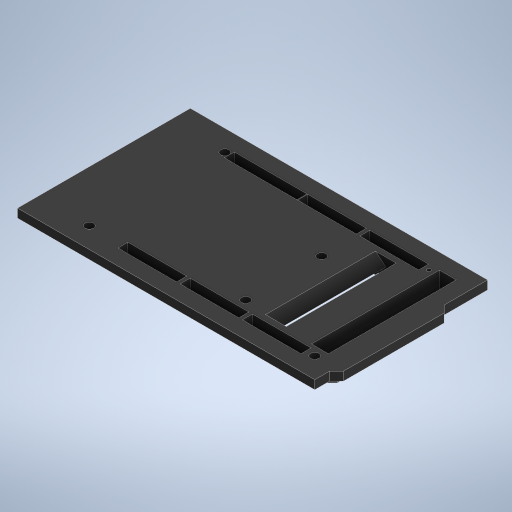
# Autodesk Inventor part: ArduinoMegaCaseTop
Saved by Autodesk Inventor 2024 (Build 280153000, 153)
## iProperties
Created: 2023-07-08
Part Number: ArduinoMegaCaseTop
Material: Rubber, Silicone
Document SubType Name: Modeling
Designer: 18179
Density: 1.25 g/cm^3
Appearance: Rubber - Black
Author: 18179
Autodesk Inventor part; units mm, degrees
ref_plane "YZ Plane" through (0, 0, 0) normal (1, 0, 0) x (0, 1, 0)
ref_plane "XZ Plane" through (0, 0, 0) normal (0, 1, 0) x (-1, 0, 0)
ref_plane "XY Plane" through (0, 0, 0) normal (0, 0, 1) x (1, 0, 0)
sketch "Sketch3" plane through (0, 0, 0) normal (0, 1, 0) x (-1, 0, 0)
  line L0 (0, 0) -> (0, -53.34)
  line L1 (0, -53.34) -> (0, -50.165)
  line L2 (0, -50.165) -> (1.905, -50.165)
  line L3 (1.905, -50.165) -> (0, -50.165)
  line L4 (0, -50.165) -> (0, -41.165)
  line L5 (0, -41.165) -> (1.905, -41.165)
  line L6 (1.905, -41.165) -> (1.905, -50.165)
  line L7 (0, 0) -> (0, -9.3)
  line L8 (0, -9.3) -> (6.35, -9.3)
  line L9 (6.35, -9.3) -> (0, -9.3)
  line L10 (0, -9.3) -> (0, -21.34)
  line L11 (0, -21.34) -> (6.35, -21.34)
  line L12 (6.35, -21.34) -> (6.35, -9.3)
  line L13 (0, -53.34) -> (-99.06, -53.34)
  line L14 (0, 0) -> (-99.06, 0)
  line L15 (0, -53.34) -> (-13.67, -53.34) construction
  line L16 (-13.67, -53.34) -> (-13.67, -50.8) construction
  line L17 (-13.67, -50.8) -> (0, -50.8) construction
  line L18 (0, -50.8) -> (0, -53.34) construction
  line L19 (0, 0) -> (-15.24, 0) construction
  line L20 (-15.24, 0) -> (-15.24, -2.54) construction
  line L21 (-15.24, -2.54) -> (0, -2.54) construction
  line L22 (0, -2.54) -> (0, 0) construction
  line L23 (-99.06, 0) -> (-90.17, 0) construction
  line L24 (-90.17, 0) -> (-90.17, -2.54) construction
  line L25 (-90.17, -2.54) -> (-99.06, -2.54) construction
  line L26 (-99.06, -2.54) -> (-99.06, 0) construction
  line L27 (-99.06, -53.34) -> (-96.52, -53.34) construction
  line L28 (-96.52, -53.34) -> (-96.52, -50.8) construction
  line L29 (-96.52, -50.8) -> (-99.06, -50.8) construction
  line L30 (-99.06, -50.8) -> (-99.06, -53.34) construction
  line L31 (-99.06, 0) -> (-66.04, 0) construction
  line L32 (-66.04, 0) -> (-66.04, -17.78) construction
  line L33 (-66.04, -17.78) -> (-99.06, -17.78) construction
  line L34 (-99.06, -17.78) -> (-99.06, 0) construction
  line L35 (-99.06, -53.34) -> (-66.04, -53.34) construction
  line L36 (-66.04, -53.34) -> (-66.04, -45.72) construction
  line L37 (-66.04, -45.72) -> (-99.06, -45.72) construction
  line L38 (-99.06, -45.72) -> (-99.06, -53.34) construction
  line L39 (-99.06, 0) -> (-99.06, -12.954)
  line L40 (-99.06, -53.34) -> (-99.06, -50.8)
  line L41 (-99.06, -50.8) -> (-101.6, -50.8) construction
  line L42 (-101.6, -50.8) -> (-101.6, -48.26) construction
  line L43 (-101.6, -48.26) -> (-99.06, -48.26) construction
  line L44 (-99.06, -48.26) -> (-99.06, -50.8) construction
  line L45 (-99.06, -12.954) -> (-101.6, -12.954) construction
  line L46 (-101.6, -12.954) -> (-101.6, -15.494) construction
  line L47 (-101.6, -15.494) -> (-99.06, -15.494) construction
  line L48 (-99.06, -15.494) -> (-99.06, -12.954) construction
  line L49 (-99.06, -12.954) -> (-101.6, -15.494)
  line L50 (-101.6, -15.494) -> (-101.6, -48.26)
  line L51 (-101.6, -48.26) -> (-99.06, -50.8)
  circle A0 centre (-13.67, -50.8) radius 1.5875
  circle A1 centre (-15.24, -2.54) radius 1.5875
  circle A2 centre (-66.04, -17.78) radius 1.5875
  circle A3 centre (-66.04, -45.72) radius 1.5875
  circle A4 centre (-96.52, -50.8) radius 1.5875
  circle A5 centre (-90.17, -2.54) radius 1.5875
  line L52 (0, -58.42) -> (-104.14, -58.42)
  line L53 (-104.14, -58.42) -> (-104.14, -52.9042)
  line L54 (-104.14, -52.9042) -> (-106.68, -50.3642)
  line L55 (-106.68, -50.3642) -> (-106.68, -13.3898)
  line L56 (-106.68, -13.3898) -> (-104.14, -10.8498)
  line L57 (-104.14, -10.8498) -> (-104.14, 5.08)
  line L58 (-104.14, 5.08) -> (0, 5.08)
  line L59 (0, -55.245) -> (-100.965, -55.245)
  line L60 (-100.965, -55.245) -> (-100.965, -51.5891)
  line L61 (-100.965, -51.5891) -> (-103.505, -49.0491)
  line L62 (-103.505, -49.0491) -> (-103.505, -14.7049)
  line L63 (-103.505, -14.7049) -> (-100.965, -12.1649)
  line L64 (-100.965, -12.1649) -> (-100.965, 1.905)
  line L65 (-100.965, 1.905) -> (0, 1.905)
  line L66 (5.08, 0) -> (5.08, -53.34)
  line L67 (1.905, 0) -> (1.905, -53.34)
  line L68 (0, -58.42) -> (5.08, -58.42)
  line L69 (5.08, -58.42) -> (5.08, -53.34)
  line L70 (1.905, -53.34) -> (1.905, -55.245)
  line L71 (1.905, -55.245) -> (0, -55.245)
  line L72 (1.905, 0) -> (1.905, 1.905)
  line L73 (1.905, 1.905) -> (0, 1.905)
  line L74 (0, 5.08) -> (5.08, 5.08)
  line L75 (5.08, 5.08) -> (5.08, 0)
  line L76 (-0.5101, -40.6549) -> (-0.5101, -50.6751)
  line L77 (-0.5101, -50.6751) -> (2.4151, -50.6751)
  line L78 (2.4151, -50.6751) -> (2.4151, -40.6549)
  line L79 (2.4151, -40.6549) -> (-0.5101, -40.6549)
  line L80 (-102.9276, -14.9441) -> (-102.9276, -48.8099)
  line L81 (-102.9276, -48.8099) -> (-100.3876, -51.3499)
  line L82 (-100.3876, -51.3499) -> (-100.3876, -54.6676)
  line L83 (-100.3876, -54.6676) -> (1.3276, -54.6676)
  line L84 (1.3276, -54.6676) -> (1.3276, -53.34)
  line L85 (1.3276, -53.34) -> (1.3276, 0)
  line L86 (1.3276, 0) -> (1.3276, 1.3276)
  line L87 (1.3276, 1.3276) -> (-100.3876, 1.3276)
  line L88 (-100.3876, 1.3276) -> (-100.3876, -12.4041)
  line L89 (-100.3876, -12.4041) -> (-102.9276, -14.9441)
  line L90 (-100.3876, -51.3499) -> (-100.965, -51.5891)
  line L91 (-100.965, -12.1649) -> (-100.3876, -12.4041)
  line L92 (1.3276, -50.6751) -> (-8.8224, -50.6751)
  line L93 (-8.8224, -50.6751) -> (-8.8224, -40.6549)
  line L94 (-8.8224, -40.6549) -> (1.3276, -40.6549)
  line L95 (1.3276, -40.6549) -> (1.3276, -50.6751)
  line L96 (0, -9.3) -> (-12.595, -9.3)
  line L97 (-12.595, -9.3) -> (-12.595, -21.34)
  line L98 (-12.595, -21.34) -> (0, -21.34)
  line L99 (0, -21.34) -> (0, -9.3)
  line L100 (0.7276, -22.0676) -> (-13.3226, -22.0676)
  line L101 (-13.3226, -22.0676) -> (-13.3226, -8.5724)
  line L102 (-13.3226, -8.5724) -> (0.7276, -8.5724)
  line L103 (0.7276, -8.5724) -> (0.7276, -22.0676)
  point P0 (5.08, -21.34)
  point P1 (1.905, -21.34)
  point P2 (1.905, -9.3)
  point P3 (5.08, -9.3)
  point P4 (0.7276, -9.3)
  point P5 (1.3276, -9.3)
  point P6 (1.3276, -40.6549)
  point P7 (1.3276, -21.34)
  point P8 (0.7276, -21.34)
  dimension "d74" = 53.34
  dimension "d75" = 3.175
  dimension "d76" = 1.905
  dimension "d77" = 9
  dimension "d78" = 9.3
  dimension "d79" = 6.35
  dimension "d80" = 12.04
  dimension "d81" = 99.06
  dimension "d82" = 99.06
  dimension "d83" = 13.67
  dimension "d84" = 2.54
  dimension "d85" = 15.24
  dimension "d86" = 2.54
  dimension "d87" = 8.89
  dimension "d88" = 2.54
  dimension "d89" = 2.54
  dimension "d90" = 2.54
  dimension "d91" = 17.78
  dimension "d92" = 33.02
  dimension "d93" = 33.02
  dimension "d94" = 7.62
  dimension "d95" = 12.954
  dimension "d96" = 2.54
  dimension "d97" = 2.54
  dimension "d98" = 2.54
  dimension "d99" = 2.54
  dimension "d100" = 2.54
  dimension "d101" = 3.175
  dimension "d102" = 3.175
  dimension "d103" = 3.175
  dimension "d104" = 3.175
  dimension "d105" = 3.175
  dimension "d106" = 3.175
  dimension "d107" = 5.08
  dimension "d108" = 3.175
  dimension "d109" = 5.08
  dimension "d110" = 3.175
  dimension "d193" = 10.15
  dimension "d194" = 12.595
  constraints: 208 end point, 31 parallel, 19 perpendicular, 16 horizontal, 9 point on line, 6 centre point, 6 coincident, 2 vertical, 1 collinear, 27 other
  measures "d74" distance of L0.start L0.end
  measures "d75" distance of L0.end L1.end
  measures "d76" distance of L1.end L2.end
  measures "d77" distance of L3.end L4.end
  measures "d78" distance of L0.start L7.end
  measures "d79" distance of L7.end L8.end
  measures "d80" distance of L10.end L9.end
  measures "d81" distance of L0.end L13.end
  measures "d82" distance of L0.start L14.end
  measures "d83" distance of L16.end L17.end
  measures "d84" distance of L15.end L16.end
  measures "d85" distance of L21.end L20.end
  measures "d86" distance of L20.end L19.end
  measures "d87" distance of L24.end L25.end
  measures "d88" distance of L23.end L24.end
  measures "d89" distance of L29.end L28.end
  measures "d90" distance of L28.end L27.end
  measures "d91" distance of L31.end L32.end
  measures "d92" distance of L32.end L33.end
  measures "d93" distance of L37.end L36.end
  measures "d94" distance of L36.end L35.end
  measures "d95" distance of L14.end L39.end
  measures "d96" distance of L13.end L29.end
  measures "d97" distance of L42.end L43.end
  measures "d98" distance of L41.end L42.end
  measures "d99" distance of L47.end L46.end
  measures "d100" distance of L46.end L45.end
  measures "d101" diameter of A0
  measures "d102" diameter of A1
  measures "d103" diameter of A2
  measures "d104" diameter of A3
  measures "d105" diameter of A4
  measures "d106" diameter of A5
  measures "d107" distance between parallel lines of L13 L52
  measures "d108" distance between parallel lines of L52 L59
  measures "d109" distance between parallel lines of L0 L66
  measures "d110" distance between parallel lines of L66 L67
  measures "d193" distance of L93.end L94.end
  measures "d194" distance of L98.end L97.end
sketch "Sketch5" plane through (0, 0, 0) normal (0, 1, 0) x (-1, 0, 0)
  line L0 (0, 0) -> (0, -53.34)
  line L1 (0, -53.34) -> (0, -50.165)
  line L2 (0, -50.165) -> (1.905, -50.165)
  line L3 (1.905, -50.165) -> (0, -50.165)
  line L4 (0, -50.165) -> (0, -41.165)
  line L5 (0, -41.165) -> (1.905, -41.165)
  line L6 (1.905, -41.165) -> (1.905, -50.165)
  line L7 (0, 0) -> (0, -9.3)
  line L8 (0, -9.3) -> (6.35, -9.3)
  line L9 (6.35, -9.3) -> (0, -9.3)
  line L10 (0, -9.3) -> (0, -21.34)
  line L11 (0, -21.34) -> (6.35, -21.34)
  line L12 (6.35, -21.34) -> (6.35, -9.3)
  line L13 (0, -53.34) -> (-99.06, -53.34)
  line L14 (0, 0) -> (-99.06, 0)
  line L15 (0, -53.34) -> (-13.67, -53.34) construction
  line L16 (-13.67, -53.34) -> (-13.67, -50.8) construction
  line L17 (-13.67, -50.8) -> (0, -50.8) construction
  line L18 (0, -50.8) -> (0, -53.34) construction
  line L19 (0, 0) -> (-15.24, 0) construction
  line L20 (-15.24, 0) -> (-15.24, -2.54) construction
  line L21 (-15.24, -2.54) -> (0, -2.54) construction
  line L22 (0, -2.54) -> (0, 0) construction
  line L23 (-99.06, 0) -> (-90.17, 0) construction
  line L24 (-90.17, 0) -> (-90.17, -2.54) construction
  line L25 (-90.17, -2.54) -> (-99.06, -2.54) construction
  line L26 (-99.06, -2.54) -> (-99.06, 0) construction
  line L27 (-99.06, -53.34) -> (-96.52, -53.34) construction
  line L28 (-96.52, -53.34) -> (-96.52, -50.8) construction
  line L29 (-96.52, -50.8) -> (-99.06, -50.8) construction
  line L30 (-99.06, -50.8) -> (-99.06, -53.34) construction
  line L31 (-99.06, 0) -> (-66.04, 0) construction
  line L32 (-66.04, 0) -> (-66.04, -17.78) construction
  line L33 (-66.04, -17.78) -> (-99.06, -17.78) construction
  line L34 (-99.06, -17.78) -> (-99.06, 0) construction
  line L35 (-99.06, -53.34) -> (-66.04, -53.34) construction
  line L36 (-66.04, -53.34) -> (-66.04, -45.72) construction
  line L37 (-66.04, -45.72) -> (-99.06, -45.72) construction
  line L38 (-99.06, -45.72) -> (-99.06, -53.34) construction
  line L39 (-99.06, 0) -> (-99.06, -12.954)
  line L40 (-99.06, -53.34) -> (-99.06, -50.8)
  line L41 (-99.06, -50.8) -> (-101.6, -50.8) construction
  line L42 (-101.6, -50.8) -> (-101.6, -48.26) construction
  line L43 (-101.6, -48.26) -> (-99.06, -48.26) construction
  line L44 (-99.06, -48.26) -> (-99.06, -50.8) construction
  line L45 (-99.06, -12.954) -> (-101.6, -12.954) construction
  line L46 (-101.6, -12.954) -> (-101.6, -15.494) construction
  line L47 (-101.6, -15.494) -> (-99.06, -15.494) construction
  line L48 (-99.06, -15.494) -> (-99.06, -12.954) construction
  line L49 (-99.06, -12.954) -> (-101.6, -15.494)
  line L50 (-101.6, -15.494) -> (-101.6, -48.26)
  line L51 (-101.6, -48.26) -> (-99.06, -50.8)
  circle A0 centre (-13.67, -50.8) radius 1.5875
  circle A1 centre (-15.24, -2.54) radius 1.5875
  circle A2 centre (-66.04, -17.78) radius 1.5875
  circle A3 centre (-66.04, -45.72) radius 1.5875
  circle A4 centre (-96.52, -50.8) radius 1.5875
  circle A5 centre (-90.17, -2.54) radius 1.5875
  line L52 (0, -58.42) -> (-104.14, -58.42)
  line L53 (-104.14, -58.42) -> (-104.14, -52.9042)
  line L54 (-104.14, -52.9042) -> (-106.68, -50.3642)
  line L55 (-106.68, -50.3642) -> (-106.68, -13.3898)
  line L56 (-106.68, -13.3898) -> (-104.14, -10.8498)
  line L57 (-104.14, -10.8498) -> (-104.14, 5.08)
  line L58 (-104.14, 5.08) -> (0, 5.08)
  line L59 (0, -55.245) -> (-100.965, -55.245)
  line L60 (-100.965, -55.245) -> (-100.965, -51.5891)
  line L61 (-100.965, -51.5891) -> (-103.505, -49.0491)
  line L62 (-103.505, -49.0491) -> (-103.505, -14.7049)
  line L63 (-103.505, -14.7049) -> (-100.965, -12.1649)
  line L64 (-100.965, -12.1649) -> (-100.965, 1.905)
  line L65 (-100.965, 1.905) -> (0, 1.905)
  line L66 (5.08, 0) -> (5.08, -53.34)
  line L67 (1.905, 0) -> (1.905, -53.34)
  line L68 (0, -58.42) -> (5.08, -58.42)
  line L69 (5.08, -58.42) -> (5.08, -53.34)
  line L70 (1.905, -53.34) -> (1.905, -55.245)
  line L71 (1.905, -55.245) -> (0, -55.245)
  line L72 (1.905, 0) -> (1.905, 1.905)
  line L73 (1.905, 1.905) -> (0, 1.905)
  line L74 (0, 5.08) -> (5.08, 5.08)
  line L75 (5.08, 5.08) -> (5.08, 0)
  dimension "d148" = 53.34
  dimension "d149" = 3.175
  dimension "d150" = 1.905
  dimension "d151" = 9
  dimension "d152" = 9.3
  dimension "d153" = 6.35
  dimension "d154" = 12.04
  dimension "d155" = 99.06
  dimension "d156" = 99.06
  dimension "d157" = 13.67
  dimension "d158" = 2.54
  dimension "d159" = 15.24
  dimension "d160" = 2.54
  dimension "d161" = 8.89
  dimension "d162" = 2.54
  dimension "d163" = 2.54
  dimension "d164" = 2.54
  dimension "d165" = 17.78
  dimension "d166" = 33.02
  dimension "d167" = 33.02
  dimension "d168" = 7.62
  dimension "d169" = 12.954
  dimension "d170" = 2.54
  dimension "d171" = 2.54
  dimension "d172" = 2.54
  dimension "d173" = 2.54
  dimension "d174" = 2.54
  dimension "d175" = 3.175
  dimension "d176" = 3.175
  dimension "d177" = 3.175
  dimension "d178" = 3.175
  dimension "d179" = 3.175
  dimension "d180" = 3.175
  dimension "d181" = 5.08
  dimension "d182" = 3.175
  dimension "d183" = 5.08
  dimension "d184" = 3.175
  constraints: 152 end point, 23 parallel, 15 perpendicular, 14 horizontal, 7 point on line, 6 centre point, 6 coincident, 2 vertical, 1 collinear, 12 other
  measures "d148" distance of L0.start L0.end
  measures "d149" distance of L0.end L1.end
  measures "d150" distance of L1.end L2.end
  measures "d151" distance of L3.end L4.end
  measures "d152" distance of L0.start L7.end
  measures "d153" distance of L7.end L8.end
  measures "d154" distance of L10.end L9.end
  measures "d155" distance of L0.end L13.end
  measures "d156" distance of L0.start L14.end
  measures "d157" distance of L16.end L17.end
  measures "d158" distance of L15.end L16.end
  measures "d159" distance of L21.end L20.end
  measures "d160" distance of L20.end L19.end
  measures "d161" distance of L24.end L25.end
  measures "d162" distance of L23.end L24.end
  measures "d163" distance of L29.end L28.end
  measures "d164" distance of L28.end L27.end
  measures "d165" distance of L31.end L32.end
  measures "d166" distance of L32.end L33.end
  measures "d167" distance of L37.end L36.end
  measures "d168" distance of L36.end L35.end
  measures "d169" distance of L14.end L39.end
  measures "d170" distance of L13.end L29.end
  measures "d171" distance of L42.end L43.end
  measures "d172" distance of L41.end L42.end
  measures "d173" distance of L47.end L46.end
  measures "d174" distance of L46.end L45.end
  measures "d175" diameter of A0
  measures "d176" diameter of A1
  measures "d177" diameter of A2
  measures "d178" diameter of A3
  measures "d179" diameter of A4
  measures "d180" diameter of A5
  measures "d181" distance between parallel lines of L13 L52
  measures "d182" distance between parallel lines of L52 L59
  measures "d183" distance between parallel lines of L0 L66
  measures "d184" distance between parallel lines of L66 L67
extrude "Extrusion1" add sketch "Sketch5" against normal blind 3.175 contours L14 L39 L49 L50 L51 L40 L13 L0 L2 L67 L70 L71 L59 L60 L61 L62 L63 L64 L65 L73 L72 L8 | L0 L13 L40 L51 L50 L49 L39 L14 | L8 L67 L11 L0 | L11 L67 L5 L0 | L67 L72 L73 L65 L64 L63 L62 L61 L60 L59 L71 L70 L6 L11 L66 L69 L68 L52 L53 L54 L55 L56 L57 L58 L74 L75 L8 | L8 L66 L11 L67 | L5 L6 L2 L0
extrude "Extrusion5" add sketch "Sketch3" against normal blind 6.35 contours L102 L101 L100 L0 L79 L94 L93 L92 L77 L13 L40 L51 L50 L49 L39 L14 | L0 L14 L39 L49 L50 L51 L40 L13 L77 L85 L84 L83 L82 L81 L80 L89 L88 L87 L86 L8 L103 L102 | L100 L103 L11 L85 L79 L0
sketch "Sketch12" plane through (0, 0, 0) normal (0, 1, 0) x (1, 0, 0)
  circle A0 centre (90.17, 2.54) radius 1.5875 projected
  circle A1 centre (96.52, 50.8) radius 1.5875 projected
  circle A2 centre (66.04, 45.72) radius 1.5875 projected
  circle A3 centre (66.04, 17.78) radius 1.5875 projected
  circle A4 centre (15.24, 2.54) radius 1.5875 projected
  circle A5 centre (13.67, 50.8) radius 1.5875 projected
  line L0 (-5.08, 58.42) -> (-5.08, -5.08) projected
  line L1 (-5.08, -5.08) -> (104.14, -5.08) projected
  line L2 (104.14, -5.08) -> (104.14, 10.8498) projected
  line L3 (104.14, 10.8498) -> (106.68, 13.3898) projected
  line L4 (106.68, 13.3898) -> (106.68, 50.3642) projected
  line L5 (106.68, 50.3642) -> (104.14, 52.9042) projected
  line L6 (104.14, 52.9042) -> (104.14, 58.42) projected
  line L7 (104.14, 58.42) -> (-5.08, 58.42) projected
  line L8 (0, 53.34) -> (0, 0)
  line L9 (0, 0) -> (99.06, 0)
  line L10 (99.06, 0) -> (99.06, 12.954)
  line L11 (99.06, 12.954) -> (101.6, 15.494)
  line L12 (101.6, 15.494) -> (101.6, 48.26)
  line L13 (101.6, 48.26) -> (99.06, 50.8)
  line L14 (99.06, 50.8) -> (99.06, 53.34)
  line L15 (99.06, 53.34) -> (0, 53.34)
  line L16 (0, 0) -> (17.526, 0)
  line L17 (17.526, 0) -> (17.526, 1.335)
  line L18 (17.526, 1.335) -> (0, 1.335)
  line L19 (0, 1.335) -> (0, 0)
  line L20 (17.526, 1.335) -> (42.926, 1.335)
  line L21 (42.926, 1.335) -> (42.926, 3.745)
  line L22 (42.926, 3.745) -> (17.526, 3.745)
  line L23 (17.526, 3.745) -> (17.526, 1.335)
  line L24 (42.926, 1.335) -> (44.45, 1.335)
  line L25 (44.45, 1.335) -> (64.77, 1.335)
  line L26 (64.77, 1.335) -> (64.77, 3.745)
  line L27 (64.77, 3.745) -> (44.45, 3.745)
  line L28 (44.45, 3.745) -> (44.45, 1.335)
  line L29 (64.77, 1.335) -> (67.31, 1.335)
  line L30 (100.3876, -1.3276) -> (-1.3276, -1.3276) projected
  line L31 (67.31, 1.335) -> (87.63, 1.335)
  line L32 (87.63, 1.335) -> (87.63, 3.745)
  line L33 (87.63, 3.745) -> (67.31, 3.745)
  line L34 (67.31, 3.745) -> (67.31, 1.335)
  line L35 (0, 53.34) -> (26.67, 53.34)
  line L36 (26.67, 53.34) -> (26.67, 52.005)
  line L37 (26.67, 52.005) -> (0, 52.005)
  line L38 (0, 52.005) -> (0, 53.34)
  line L39 (26.67, 52.005) -> (46.99, 52.005)
  line L40 (46.99, 52.005) -> (46.99, 49.595)
  line L41 (46.99, 49.595) -> (26.67, 49.595)
  line L42 (26.67, 49.595) -> (26.67, 52.005)
  line L43 (46.99, 52.005) -> (49.53, 52.005)
  line L44 (48.9034, 50.8262) -> (49.53, 52.005)
  line L45 (49.53, 52.005) -> (69.85, 52.005)
  line L46 (69.85, 52.005) -> (69.85, 49.595)
  line L47 (69.85, 49.595) -> (49.53, 49.595)
  line L48 (49.53, 49.595) -> (49.53, 52.005)
  line L49 (69.85, 52.005) -> (72.39, 52.005)
  line L50 (72.39, 52.005) -> (92.71, 52.005)
  line L51 (92.71, 52.005) -> (92.71, 49.595)
  line L52 (92.71, 49.595) -> (72.39, 49.595)
  line L53 (72.39, 49.595) -> (72.39, 52.005)
  line L54 (92.71, 49.595) -> (92.775, 49.595)
  line L55 (92.775, 49.595) -> (92.775, 46.99)
  line L56 (92.775, 46.99) -> (92.71, 46.99)
  line L57 (92.71, 46.99) -> (92.71, 49.595)
  line L58 (92.775, 46.99) -> (97.725, 46.99)
  line L59 (97.725, 46.99) -> (97.725, 1.27)
  line L60 (97.725, 1.27) -> (92.775, 1.27)
  line L61 (92.775, 1.27) -> (92.775, 46.99)
  point P0 (0, 0)
  dimension "d236" = 5.08
  dimension "d237" = 17.526
  dimension "d238" = 1.335
  dimension "d239" = 25.4
  dimension "d240" = 2.41
  dimension "d241" = 1.524
  dimension "d242" = 20.32
  dimension "d243" = 2.54
  dimension "d244" = 20.32
  dimension "d245" = 26.67
  dimension "d246" = 1.335
  dimension "d247" = 20.32
  dimension "d248" = 2.41
  dimension "d249" = 2.54
  dimension "d250" = 1.335
  dimension "d251" = 20.32
  dimension "d252" = 2.41
  dimension "d253" = 2.54
  dimension "d254" = 20.32
  dimension "d255" = 0.065
  dimension "d256" = 2.605
  dimension "d257" = 4.95
  dimension "d258" = 45.72
  constraints: 106 end point, 21 parallel, 13 horizontal, 10 perpendicular, 1 point on line, 7 other
  measures "d236" distance between parallel lines of L7 L15
  measures "d237" distance of L18.end L17.end
  measures "d238" distance of L17.end L16.end
  measures "d239" distance of L22.end L21.end
  measures "d240" distance of L21.end L20.end
  measures "d241" distance of L20.end L24.end
  measures "d242" distance of L27.end L26.end
  measures "d243" distance of L25.end L29.end
  measures "d244" distance of L33.end L32.end
  measures "d245" distance of L36.end L37.end
  measures "d246" distance of L35.end L36.end
  measures "d247" distance of L40.end L41.end
  measures "d248" distance of L39.end L40.end
  measures "d249" distance of L39.end L43.end
  measures "d250" distance of L43.end L44.start
  measures "d251" distance of L47.start L47.end
  measures "d252" distance of L49.start L47.start
  measures "d253" distance of L49.start L49.end
  measures "d254" distance of L51.end L52.end
  measures "d255" distance of L55.end L56.end
  measures "d256" distance of L54.end L55.end
  measures "d257" distance of L59.end L60.end
  measures "d258" distance of L58.end L59.end
extrude "Extrusion6" cut sketch "Sketch12" against normal blind 6.35 contours L23 L22 L21 L20 | L39 L40 L41 L42 | L28 L27 L26 L25 | L34 L33 L32 L31 | L45 L46 L47 L48 | L58 L59 L60 L61 | L50 L51 L52 L53
sketch "Sketch13" plane through (0, -6.35, 0) normal (0, -1, 0) x (1, 0, 0)
  line L0 (-0.7276, -9.3) -> (-0.7276, -8.5724) projected
  line L1 (-1.3276, 1.3276) -> (-1.3276, -9.3) projected
  line L2 (-0.7276, -8.5724) -> (-1.3276, -8.5724)
  line L3 (-1.3276, -8.5724) -> (-1.3276, -9.3)
  line L4 (-1.3276, -9.3) -> (-0.7276, -9.3)
  line L5 (-0.7276, -9.3) -> (-0.7276, -8.5724)
  line L6 (-0.7276, -22.0676) -> (-0.7276, -21.34) projected
  line L7 (-1.3276, -21.34) -> (-1.3276, -40.6549) projected
  line L8 (-0.7276, -22.0676) -> (-1.3276, -22.0676)
  line L9 (-1.3276, -22.0676) -> (-1.3276, -21.34)
  line L10 (-1.3276, -21.34) -> (-0.7276, -21.34)
  line L11 (-0.7276, -21.34) -> (-0.7276, -22.0676)
  point P0 (0, 0)
  constraints: 16 end point, 4 parallel, 2 horizontal, 2 perpendicular
extrude "Extrusion7" cut sketch "Sketch13" against normal up to surface (3.175 mm away)
sketch "Sketch14" plane through (0, -6.35, 0) normal (0, -1, 0) x (1, 0, 0)
  line L0 (8.8224, -40.6549) -> (-1.3276, -40.6549) projected
  line L1 (8.8224, -40.6549) -> (12.5371, -40.6549)
  line L2 (12.5371, -40.6549) -> (12.5371, -50.6751)
  line L3 (12.5371, -50.6751) -> (8.8224, -50.6751)
  line L4 (8.8224, -50.6751) -> (8.8224, -40.6549)
  point P0 (0, 0)
  constraints: 8 end point, 2 parallel, 1 horizontal, 1 perpendicular
extrude "Extrusion8" cut sketch "Sketch14" against normal up to surface (3.175 mm away)
mirror "Mirror1" about plane through (104.14, 0, 5.08) normal (0, 0, 1) remove original yes
sketch "Sketch15" plane through (-5.08, 0, 68.58) normal (0, 1, 0) x (1, 0, 0)
  line L0 (72.39, 54.675) -> (92.71, 54.675) projected
  line L1 (72.39, 57.085) -> (72.39, 54.675) projected
  line L2 (92.71, 57.085) -> (72.39, 57.085) projected
  line L3 (92.71, 54.675) -> (92.71, 57.085) projected
  line L4 (97.79, 6.415) -> (97.79, 8.825) projected
  line L5 (77.47, 6.415) -> (97.79, 6.415) projected
  line L6 (77.47, 8.825) -> (77.47, 6.415) projected
  line L7 (97.79, 8.825) -> (77.47, 8.825) projected
  line L8 (102.805, 11.43) -> (102.805, 57.15) projected
  line L9 (97.855, 11.43) -> (102.805, 11.43) projected
  line L10 (97.855, 57.15) -> (97.855, 11.43) projected
  line L11 (102.805, 57.15) -> (97.855, 57.15) projected
  line L12 (49.53, 54.675) -> (69.85, 54.675) projected
  line L13 (49.53, 57.085) -> (49.53, 54.675) projected
  line L14 (69.85, 57.085) -> (49.53, 57.085) projected
  line L15 (69.85, 54.675) -> (69.85, 57.085) projected
  line L16 (74.93, 6.415) -> (74.93, 8.825) projected
  line L17 (54.61, 6.415) -> (74.93, 6.415) projected
  line L18 (54.61, 8.825) -> (54.61, 6.415) projected
  line L19 (74.93, 8.825) -> (54.61, 8.825) projected
  line L20 (52.07, 6.415) -> (52.07, 8.825) projected
  line L21 (31.75, 6.415) -> (52.07, 6.415) projected
  line L22 (31.75, 8.825) -> (31.75, 6.415) projected
  line L23 (52.07, 8.825) -> (31.75, 8.825) projected
  line L24 (22.606, 54.675) -> (48.006, 54.675) projected
  line L25 (22.606, 57.085) -> (22.606, 54.675) projected
  line L26 (48.006, 57.085) -> (22.606, 57.085) projected
  line L27 (48.006, 54.675) -> (48.006, 57.085) projected
  circle A0 centre (95.25, 55.88) radius 1.5875 projected
  circle A1 centre (101.6, 7.62) radius 1.5875 projected
  circle A2 centre (71.12, 12.7) radius 1.5875 projected
  circle A3 centre (71.12, 40.64) radius 1.5875 projected
  circle A4 centre (20.32, 55.88) radius 1.5875 projected
  circle A5 centre (18.75, 7.62) radius 1.5875 projected
  line L28 (0, 0) -> (0, 63.5) projected
  line L29 (109.22, 0) -> (0, 0) projected
  line L30 (109.22, 5.5158) -> (109.22, 0) projected
  line L31 (111.76, 8.0558) -> (109.22, 5.5158) projected
  line L32 (111.76, 45.0302) -> (111.76, 8.0558) projected
  line L33 (109.22, 47.5702) -> (111.76, 45.0302) projected
  line L34 (109.22, 63.5) -> (109.22, 47.5702) projected
  line L35 (0, 63.5) -> (109.22, 63.5) projected
  line L36 (97.22, 10.795) -> (103.44, 10.795)
  line L37 (103.44, 10.795) -> (103.44, 57.785)
  line L38 (103.44, 57.785) -> (97.22, 57.785)
  line L39 (97.22, 57.785) -> (97.22, 10.795)
  line L40 (76.835, 9.46) -> (76.835, 5.78)
  line L41 (76.835, 5.78) -> (98.425, 5.78)
  line L42 (98.425, 5.78) -> (98.425, 9.46)
  line L43 (98.425, 9.46) -> (76.835, 9.46)
  line L44 (53.975, 9.46) -> (53.975, 5.78)
  line L45 (53.975, 5.78) -> (75.565, 5.78)
  line L46 (75.565, 5.78) -> (75.565, 9.46)
  line L47 (75.565, 9.46) -> (53.975, 9.46)
  line L48 (31.115, 9.46) -> (31.115, 5.78)
  line L49 (31.115, 5.78) -> (52.705, 5.78)
  line L50 (52.705, 5.78) -> (52.705, 9.46)
  line L51 (52.705, 9.46) -> (31.115, 9.46)
  line L52 (47.371, 56.45) -> (23.241, 56.45)
  line L53 (23.241, 56.45) -> (23.241, 55.31)
  line L54 (23.241, 55.31) -> (47.371, 55.31)
  line L55 (47.371, 55.31) -> (47.371, 56.45)
  line L56 (48.641, 57.72) -> (21.971, 57.72)
  line L57 (21.971, 57.72) -> (21.971, 54.04)
  line L58 (21.971, 54.04) -> (48.641, 54.04)
  line L59 (48.641, 54.04) -> (48.641, 57.72)
  line L60 (48.895, 57.72) -> (48.895, 54.04)
  line L61 (48.895, 54.04) -> (70.485, 54.04)
  line L62 (70.485, 54.04) -> (70.485, 57.72)
  line L63 (70.485, 57.72) -> (48.895, 57.72)
  line L64 (71.755, 57.72) -> (71.755, 54.04)
  line L65 (71.755, 54.04) -> (93.345, 54.04)
  line L66 (93.345, 54.04) -> (93.345, 57.72)
  line L67 (93.345, 57.72) -> (71.755, 57.72)
  point P0 (5.08, 68.58)
  dimension "d265" = 0.635
  dimension "d266" = 0.635
  dimension "d267" = 0.635
  dimension "d268" = 0.635
  dimension "d269" = 0.635
  dimension "d270" = 0.635
  dimension "d271" = 0.635
  dimension "d272" = 0.635
  constraints: 64 end point, 24 other
  measures "d265" distance between parallel lines of L10 L39
  measures "d266" distance between parallel lines of L7 L43
  measures "d267" distance between parallel lines of L19 L47
  measures "d268" distance between parallel lines of L23 L51
  measures "d269" distance between parallel lines of L27 L55
  measures "d270" distance between parallel lines of L27 L59
  measures "d271" distance between parallel lines of L14 L63
  measures "d272" distance between parallel lines of L2 L67
extrude "Extrusion9" cut sketch "Sketch15" against normal blind 25.4 contours L1 L2 L3 L0 | L5 L6 L7 L4 | L9 L10 L11 L8 | L13 L14 L15 L12 | L17 L18 L19 L16 | L21 L22 L23 L20 | L25 L26 L27 L24 | L39 L38 L37 L36 | L43 L42 L41 L40 | L47 L46 L45 L44 | L51 L50 L49 L48 | L55 L54 L53 L52 | L59 L58 L57 L56 | L63 L62 L61 L60 | L67 L66 L65 L64
sketch "Sketch16" plane through (-5.08, 0, 68.58) normal (0, 1, 0) x (1, 0, 0)
  line L0 (75.565, 9.46) -> (75.565, 5.78) projected
  line L1 (75.565, 5.78) -> (53.975, 5.78) projected
  line L2 (53.975, 5.78) -> (53.975, 9.46) projected
  line L3 (53.975, 9.46) -> (75.565, 9.46) projected
  line L4 (97.22, 57.785) -> (103.44, 57.785) projected
  line L5 (103.44, 57.785) -> (103.44, 10.795) projected
  line L6 (103.44, 10.795) -> (97.22, 10.795) projected
  line L7 (97.22, 10.795) -> (97.22, 57.785) projected
  line L8 (70.485, 57.72) -> (70.485, 54.04) projected
  line L9 (70.485, 54.04) -> (48.895, 54.04) projected
  line L10 (48.895, 54.04) -> (48.895, 57.72) projected
  line L11 (48.895, 57.72) -> (70.485, 57.72) projected
  line L12 (52.705, 9.46) -> (52.705, 5.78) projected
  line L13 (52.705, 5.78) -> (31.115, 5.78) projected
  line L14 (31.115, 5.78) -> (31.115, 9.46) projected
  line L15 (31.115, 9.46) -> (52.705, 9.46) projected
  line L16 (98.425, 9.46) -> (98.425, 5.78) projected
  line L17 (98.425, 5.78) -> (76.835, 5.78) projected
  line L18 (76.835, 5.78) -> (76.835, 9.46) projected
  line L19 (76.835, 9.46) -> (98.425, 9.46) projected
  line L20 (93.345, 57.72) -> (93.345, 54.04) projected
  line L21 (93.345, 54.04) -> (71.755, 54.04) projected
  line L22 (71.755, 54.04) -> (71.755, 57.72) projected
  line L23 (71.755, 57.72) -> (93.345, 57.72) projected
  line L24 (48.641, 54.04) -> (21.971, 54.04) projected
  line L25 (21.971, 54.04) -> (21.971, 57.72) projected
  line L26 (21.971, 57.72) -> (48.641, 57.72) projected
  line L27 (48.641, 57.72) -> (48.641, 54.04) projected
  circle A0 centre (95.25, 55.88) radius 1.5875 projected
  circle A1 centre (101.6, 7.62) radius 1.5875 projected
  circle A2 centre (71.12, 12.7) radius 1.5875 projected
  circle A3 centre (71.12, 40.64) radius 1.5875 projected
  circle A4 centre (20.32, 55.88) radius 1.5875 projected
  circle A5 centre (18.75, 7.62) radius 1.5875 projected
  line L28 (0, 0) -> (0, 63.5) projected
  line L29 (109.22, 0) -> (0, 0) projected
  line L30 (109.22, 5.5158) -> (109.22, 0) projected
  line L31 (111.76, 8.0558) -> (109.22, 5.5158) projected
  line L32 (111.76, 45.0302) -> (111.76, 8.0558) projected
  line L33 (109.22, 47.5702) -> (111.76, 45.0302) projected
  line L34 (109.22, 63.5) -> (109.22, 47.5702) projected
  line L35 (0, 63.5) -> (109.22, 63.5) projected
  circle A6 centre (95.25, 55.88) radius 0.75
  point P0 (5.08, 68.58)
  dimension "d275" = 1.5
  constraints: 1 centre point, 1 coincident
  measures "d275" diameter of A6
extrude "Extrusion10" add sketch "Sketch16" against normal up to surface (6.35 mm away) contours A0
sketch "Sketch17" plane through (-5.08, 0, 68.58) normal (0, 0, 1) x (1, 0, 0)
  line L0 (97.22, 0) -> (87.06, 0)
  line L1 (87.06, 0) -> (79.44, 0)
  line L2 (79.44, 0) -> (83.0478, -3.0273)
  line L3 (87.06, 0) -> (91.9356, -4.0911)
  line L4 (91.9356, -4.0911) -> (95.0817, -6.731)
  line L5 (83.0478, -3.0273) -> (87.4617, -6.731)
  line L6 (87.4617, -6.731) -> (95.0817, -6.731)
  point P0 (5.08, 0)
  dimension "d278" = 10.16
  dimension "d279" = 7.62
  dimension "d280" = 40
  constraints: 14 end point, 2 horizontal, 2 point on line
  measures "d278" distance of L0.start L0.end
  measures "d279" distance of L0.end L1.end
  measures "d280" angle of L2 L1
extrude "Extrusion11" cut sketch "Sketch17" against normal up to surface (57.72 mm away)
sketch "Sketch18" plane through (-5.08, 0, 5.08) normal (0, 1, 0) x (1, 0, 0)
  line L0 (97.22, -52.705) -> (97.22, -5.715) projected
  line L1 (53.975, -54.04) -> (75.565, -54.04) projected
  line L2 (97.22, -52.705) -> (75.565, -52.705)
  line L3 (75.565, -52.705) -> (75.565, -54.04)
  line L4 (75.565, -54.04) -> (97.22, -54.04)
  line L5 (97.22, -54.04) -> (97.22, -52.705)
  line L6 (98.425, -57.72) -> (87.06, -57.72) projected
  line L7 (79.44, -63.5) -> (0, -63.5) projected
  line L8 (87.06, -57.72) -> (79.44, -57.72)
  line L9 (79.44, -57.72) -> (79.44, -63.5)
  line L10 (79.44, -63.5) -> (87.06, -63.5)
  line L11 (87.06, -63.5) -> (87.06, -57.72)
  line L12 (75.565, -52.705) -> (87.06, -52.705)
  line L13 (87.06, -52.705) -> (87.06, -51.8209)
  line L14 (87.06, -51.8209) -> (75.565, -51.8209)
  line L15 (75.565, -51.8209) -> (75.565, -52.705)
  line L16 (87.06, -9.46) -> (87.06, -54.04) projected
  line L17 (79.44, -63.5) -> (79.44, -9.46) projected
  line L18 (87.06, -9.46) -> (79.44, -9.46)
  line L19 (79.44, -9.46) -> (79.44, -2.0144)
  line L20 (79.44, -2.0144) -> (87.06, -2.0144)
  line L21 (87.06, -2.0144) -> (87.06, -9.46)
  line L22 (109.22, -63.5) -> (87.06, -63.5) projected
  line L23 (87.06, -57.72) -> (91.0915, -57.72)
  line L24 (91.0915, -57.72) -> (91.0915, -63.5)
  line L25 (91.0915, -63.5) -> (87.06, -63.5)
  line L26 (87.06, -63.5) -> (87.06, -57.72)
  line L27 (93.345, -9.46) -> (87.06, -9.46) projected
  line L28 (87.06, -2.0144) -> (93.345, -2.0144)
  line L29 (93.345, -2.0144) -> (93.345, -9.46)
  line L30 (93.345, -9.46) -> (87.06, -9.46)
  line L31 (87.06, -9.46) -> (87.06, -2.0144)
  line L32 (87.06, -51.8209) -> (97.22, -51.8209)
  line L33 (97.22, -51.8209) -> (97.22, -52.705)
  line L34 (97.22, -52.705) -> (87.06, -52.705)
  line L35 (87.06, -52.705) -> (87.06, -51.8209)
  line L36 (91.0915, -57.72) -> (97.22, -57.72)
  line L37 (97.22, -57.72) -> (97.22, -63.5)
  line L38 (97.22, -63.5) -> (91.0915, -63.5)
  line L39 (91.0915, -63.5) -> (91.0915, -57.72)
  line L40 (79.44, -9.46) -> (97.22, -9.46)
  line L41 (97.22, -9.46) -> (97.22, -11.4064)
  line L42 (97.22, -11.4064) -> (79.44, -11.4064)
  line L43 (79.44, -11.4064) -> (79.44, -9.46)
  point P0 (5.08, 5.08)
  point P1 (79.44, -9.46)
  point P2 (79.44, -51.8209)
  point P3 (79.44, -54.04)
  point P4 (97.22, -9.46)
  constraints: 72 end point, 18 parallel, 9 horizontal, 9 perpendicular, 6 point on line
extrude "Extrusion12" add sketch "Sketch18" against normal blind 6.35 contours L2 L13 L32 L0 | L5 L4 L16 L2 | L16 L4 L17 L2 | L2 L17 L14 L13 | L42 L16 L27 L40 L0 | L42 L17 L18 L16 | L37 L22 L24 L6 | L24 L22 L11 L6 | L11 L10 L9 L8
sketch "Sketch19" plane through (92.14, -6.35, 64.8276) normal (1, 0, 0) x (0, 0, -1)
  line L0 (0, 3.175) -> (0, 0) projected
  line L1 (-3.7524, 3.175) -> (0, 3.175) projected
  line L2 (-3.7524, 3.175) -> (-3.7524, 0) projected
  line L3 (0, 0) -> (-3.7524, 0) projected
  point P0 (64.8276, 6.35)
extrude "Extrusion13" cut sketch "Sketch19" against normal through all
sketch "Sketch20" plane through (-1.3276, -6.35, 64.8276) normal (0, -1, 0) x (1, 0, 0)
  line L0 (71.8126, -2.0276) -> (71.8126, -5.7076) projected
  line L1 (71.8126, -5.7076) -> (50.2226, -5.7076) projected
  line L2 (50.2226, -5.7076) -> (50.2226, -2.0276) projected
  line L3 (50.2226, -2.0276) -> (71.8126, -2.0276) projected
  line L4 (66.7326, -50.2876) -> (66.7326, -53.9676) projected
  line L5 (66.7326, -53.9676) -> (45.1426, -53.9676) projected
  line L6 (45.1426, -53.9676) -> (45.1426, -50.2876) projected
  line L7 (45.1426, -50.2876) -> (66.7326, -50.2876) projected
  line L8 (48.9526, -2.0276) -> (48.9526, -5.7076) projected
  line L9 (48.9526, -5.7076) -> (27.3626, -5.7076) projected
  line L10 (27.3626, -5.7076) -> (27.3626, -2.0276) projected
  line L11 (27.3626, -2.0276) -> (48.9526, -2.0276) projected
  line L12 (18.2186, -50.2876) -> (44.8886, -50.2876) projected
  line L13 (44.8886, -50.2876) -> (44.8886, -53.9676) projected
  line L14 (44.8886, -53.9676) -> (18.2186, -53.9676) projected
  line L15 (18.2186, -53.9676) -> (18.2186, -50.2876) projected
  circle A0 centre (16.5676, -52.1276) radius 1.5875 projected
  circle A1 centre (67.3676, -36.8876) radius 1.5875 projected
  circle A2 centre (67.3676, -8.9476) radius 1.5875 projected
  circle A3 centre (97.8476, -3.8676) radius 1.5875 projected
  line L16 (68.0026, -50.2876) -> (90.8753, -50.2876) projected
  line L17 (90.8753, -50.2876) -> (90.8753, -51.7091) projected
  arc A4 (90.8753, -52.5461) -> (90.8753, -51.7091) centre (91.4976, -52.1276) ccw projected
  line L18 (90.8753, -52.5461) -> (90.8753, -53.9676) projected
  line L19 (90.8753, -53.9676) -> (68.0026, -53.9676) projected
  line L20 (68.0026, -53.9676) -> (68.0026, -50.2876) projected
  line L21 (93.4676, -7.0426) -> (99.6876, -7.0426) projected
  line L22 (99.6876, -7.0426) -> (99.6876, -54.0326) projected
  line L23 (99.6876, -54.0326) -> (93.4676, -54.0326) projected
  line L24 (93.4676, -54.0326) -> (93.4676, -7.0426) projected
  line L25 (83.2553, -7.9268) -> (90.8753, -7.9268) projected
  line L26 (90.8753, -7.9268) -> (90.8753, -48.3412) projected
  line L27 (90.8753, -48.3412) -> (83.2553, -48.3412) projected
  line L28 (83.2553, -48.3412) -> (83.2553, -7.9268) projected
  line L29 (0, 0) -> (101.7152, 0) projected
  line L30 (0, -3.9925) -> (0, 0) projected
  line L31 (13.415, -3.9925) -> (0, -3.9925) projected
  arc A5 (13.8647, -4.9797) -> (13.415, -3.9925) centre (14.9976, -3.8676) ccw projected
  line L32 (13.8647, -14.0127) -> (13.8647, -4.9797) projected
  line L33 (0, -14.0127) -> (13.8647, -14.0127) projected
  line L34 (0, -32.6) -> (0, -14.0127) projected
  line L35 (14.6503, -32.6) -> (0, -32.6) projected
  line L36 (14.6503, -46.0953) -> (14.6503, -32.6) projected
  line L37 (0, -46.0953) -> (14.6503, -46.0953) projected
  line L38 (0, -55.9952) -> (0, -46.0953) projected
  line L39 (101.7152, -55.9952) -> (0, -55.9952) projected
  line L40 (101.7152, -42.2635) -> (101.7152, -55.9952) projected
  line L41 (104.2552, -39.7235) -> (101.7152, -42.2635) projected
  line L42 (104.2552, -5.8577) -> (104.2552, -39.7235) projected
  line L43 (101.7152, -3.3177) -> (104.2552, -5.8577) projected
  line L44 (101.7152, 0) -> (101.7152, -3.3177) projected
  line L45 (94.6726, -5.7076) -> (73.0826, -5.7076) projected
  line L46 (73.0826, -5.7076) -> (73.0826, -2.0276) projected
  line L47 (73.0826, -2.0276) -> (94.6726, -2.0276) projected
  line L48 (94.6726, -2.0276) -> (94.6726, -5.7076) projected
  line L49 (80.0803, -4.7518) -> (94.0503, -4.7518)
  line L50 (94.0503, -4.7518) -> (94.0503, -51.5162)
  line L51 (94.0503, -51.5162) -> (80.0803, -51.5162)
  line L52 (80.0803, -51.5162) -> (80.0803, -4.7518)
  line L53 (69.9076, -47.1126) -> (69.9076, -57.1426)
  line L54 (69.9076, -57.1426) -> (41.9676, -57.1426)
  line L55 (41.9676, -57.1426) -> (41.9676, -47.1126)
  line L56 (41.9676, -47.1126) -> (69.9076, -47.1126)
  line L57 (47.0476, -8.8826) -> (74.9876, -8.8826)
  line L58 (74.9876, -8.8826) -> (74.9876, 1.1474)
  line L59 (74.9876, 1.1474) -> (47.0476, 1.1474)
  line L60 (47.0476, 1.1474) -> (47.0476, -8.8826)
  line L61 (17.8253, -29.425) -> (3.175, -29.425)
  line L62 (3.175, -29.425) -> (3.175, -17.1877)
  line L63 (3.175, -17.1877) -> (17.0397, -17.1877)
  line L64 (17.0397, -17.1877) -> (17.0397, -8.1701)
  arc A6 (17.0397, -8.1701) -> (19.7095, -3.175) centre (14.9976, -3.8676) ccw
  line L65 (19.7095, -3.175) -> (98.5402, -3.175)
  line L66 (98.5402, -3.175) -> (98.5402, -4.6328)
  line L67 (98.5402, -4.6328) -> (101.0802, -7.1728)
  line L68 (101.0802, -7.1728) -> (101.0802, -38.4084)
  line L69 (101.0802, -38.4084) -> (98.5402, -40.9484)
  line L70 (98.5402, -40.9484) -> (98.5402, -52.8202)
  line L71 (98.5402, -52.8202) -> (3.175, -52.8202)
  line L72 (3.175, -52.8202) -> (3.175, -49.2703)
  line L73 (3.175, -49.2703) -> (17.8253, -49.2703)
  line L74 (17.8253, -49.2703) -> (17.8253, -29.425)
  line L75 (41.9676, -47.1126) -> (17.8253, -47.1126)
  line L76 (17.8253, -29.425) -> (17.8253, -7.6998)
  line L77 (74.9876, -8.8826) -> (80.0803, -8.8826)
  line L78 (80.0803, -8.8826) -> (80.0803, -4.7518)
  line L79 (80.0803, -4.7518) -> (74.9876, -4.7518)
  line L80 (74.9876, -4.7518) -> (74.9876, -8.8826)
  line L81 (69.9076, -47.1126) -> (80.0803, -47.1126)
  line L82 (80.0803, -47.1126) -> (80.0803, -51.5162)
  line L83 (80.0803, -51.5162) -> (69.9076, -51.5162)
  line L84 (69.9076, -51.5162) -> (69.9076, -47.1126)
  line L85 (-3.7524, 3.7524) -> (105.4676, 3.7524) projected
  line L86 (47.0476, -8.8826) -> (13.415, -8.8826)
  line L87 (13.415, -8.8826) -> (13.415, 3.7524)
  line L88 (13.415, 3.7524) -> (47.0476, 3.7524)
  line L89 (47.0476, 3.7524) -> (47.0476, -8.8826)
  point P0 (1.3276, -64.8276)
  point P1 (80.0803, -8.8826)
  point P2 (68.9538, -8.8826)
  point P3 (65.7815, -8.8826)
  point P4 (17.8253, -8.8826)
  dimension "d287" = 3.175
  dimension "d288" = 3.175
  dimension "d289" = 3.175
  dimension "d290" = 3.175
  constraints: 80 end point, 6 parallel, 5 perpendicular, 3 horizontal, 3 point on circle, 2 point on line, 1 centre point, 23 other
  measures "d287" distance between parallel lines of L28 L52
  measures "d288" distance between parallel lines of L7 L56
  measures "d289" distance between parallel lines of L1 L57
  measures "d290" distance between parallel lines of L36 L74
extrude "Extrusion14" cut sketch "Sketch20" against normal blind 3.175 contours L77 L52 L81 L56 L75 L74 L76 L86 L57 A2
sketch "Sketch21" plane through (81.9276, -6.35, 56.9009) normal (0.6427876, 0.7660444, 0) x (0.7660444, -0.6427876, 0)
  line L0 (-4.1447, 39.1859) -> (-4.1447, 0.9559) projected
  line L1 (-4.1447, 0.9559) -> (-4.9394, 0.9559) projected
  line L2 (-4.9394, 0.9559) -> (-4.9394, 39.1859) projected
  line L3 (-4.9394, 39.1859) -> (-4.1447, 39.1859) projected
  line L4 (-9.8788, 0) -> (0, 0) projected
  line L5 (0, 40.4145) -> (0, 0) projected
  line L6 (0, 40.4145) -> (-9.8788, 40.4145) projected
  line L7 (-9.8788, 0) -> (-9.8788, 40.4145) projected
  line L8 (-4.1447, 0.9559) -> (-4.9394, 0.9559)
  line L9 (-4.9394, 0.9559) -> (-4.9394, 0)
  line L10 (-4.9394, 0) -> (-4.1447, 0)
  line L11 (-4.1447, 0) -> (-4.1447, 0.9559)
  line L12 (-4.1447, 39.1859) -> (-4.9394, 39.1859)
  line L13 (-4.9394, 39.1859) -> (-4.9394, 40.4145)
  line L14 (-4.9394, 40.4145) -> (-4.1447, 40.4145)
  line L15 (-4.1447, 40.4145) -> (-4.1447, 39.1859)
  point P0 (-66.8419, 56.9009)
  point P1 (-4.9394, 0.9559)
  dimension "d74" = 53.34
  dimension "d75" = 3.175
  dimension "d76" = 1.905
  dimension "d77" = 9
  dimension "d78" = 9.3
  dimension "d79" = 6.35
  dimension "d80" = 12.04
  dimension "d81" = 99.06
  dimension "d82" = 99.06
  dimension "d83" = 13.67
  dimension "d84" = 2.54
  dimension "d85" = 15.24
  dimension "d86" = 2.54
  dimension "d87" = 8.89
  dimension "d88" = 2.54
  dimension "d89" = 2.54
  dimension "d90" = 2.54
  dimension "d91" = 17.78
  dimension "d92" = 33.02
  dimension "d93" = 33.02
  dimension "d94" = 7.62
  dimension "d95" = 12.954
  dimension "d96" = 2.54
  dimension "d97" = 2.54
  constraints: 16 end point, 4 parallel, 2 horizontal, 2 midpoint, 2 perpendicular
extrude "Extrusion15" cut sketch "Sketch21" against normal blind 5.08 contours L15 L6 L5 L4 L11 L0 | L3 L13 L6 L15 | L11 L4 L9 L1
body "Solid1"
